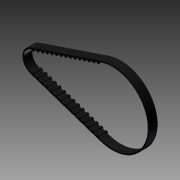
# Autodesk Inventor part: short turn belt
Saved by Autodesk Inventor 2012 (Build 160160000, 160)
## iProperties
Created: 2013-11-05
Part Number: short turn belt
Material: Default
Document SubType Name: Modeling
Designer: Bryce
Density: 1 g/cm^3
Author: Bryce
Autodesk Inventor part; units mm, degrees
ref_plane "YZ Plane" through (0, 0, 0) normal (1, 0, 0) x (0, 1, 0)
ref_plane "XZ Plane" through (0, 0, 0) normal (0, 1, 0) x (-1, 0, 0)
ref_plane "XY Plane" through (0, 0, 0) normal (0, 0, 1) x (1, 0, 0)
sketch "Sketch1" plane through (0, 0, 0) normal (0, 0, 1) x (1, 0, 0)
  arc A0 (-3.6157, 10.7627) -> (-3.6157, -10.7627) centre (0, 0) ccw
  arc A1 (70.5622, -35.683) -> (70.5622, 35.683) centre (82.55, 0) ccw
  line L0 (-3.6157, 10.7627) -> (70.5622, 35.683)
  line L1 (-3.6157, -10.7627) -> (0.5217, -12.1527)
  arc A2 (70.1335, -36.9591) -> (70.1335, 36.9591) centre (82.55, 0) ccw
  line L2 (70.1335, -36.9591) -> (-4.0445, -12.0388)
  arc A3 (-4.0445, 12.0388) -> (-4.0445, -12.0388) centre (0, 0) ccw
  line L3 (-4.0445, 12.0388) -> (70.1335, 36.9591)
  arc A4 (0.1194, -11.4488) -> (-2.8701, -10.4444) centre (-1.4338, -11.1206) ccw
  arc A5 (-3.6157, -10.7627) -> (-2.8701, -10.4444) centre (-3.4216, -10.1848) ccw
  arc A6 (0.1194, -11.4488) -> (0.5217, -12.1527) centre (0.7159, -11.5748) ccw
  line L4 (0.5217, -12.1527) -> (70.5622, -35.683)
  line L5 (1.2961, -12.4128) -> (5.4336, -13.8028)
  arc A7 (5.0313, -13.0989) -> (2.0418, -12.0946) centre (3.4781, -12.7707) ccw
  arc A8 (1.2961, -12.4128) -> (2.0418, -12.0946) centre (1.4902, -11.835) ccw
  arc A9 (5.0313, -13.0989) -> (5.4336, -13.8028) centre (5.6277, -13.225) ccw
  line L6 (6.2079, -14.063) -> (10.3454, -15.453)
  arc A10 (9.9431, -14.7491) -> (6.9536, -13.7447) centre (8.3899, -14.4209) ccw
  arc A11 (6.2079, -14.063) -> (6.9536, -13.7447) centre (6.402, -13.4851) ccw
  arc A12 (9.9431, -14.7491) -> (10.3454, -15.453) centre (10.5395, -14.8751) ccw
  line L7 (11.1197, -15.7131) -> (15.2572, -17.1031)
  arc A13 (14.8549, -16.3992) -> (11.8654, -15.3949) centre (13.3017, -16.071) ccw
  arc A14 (11.1197, -15.7131) -> (11.8654, -15.3949) centre (11.3139, -15.1352) ccw
  arc A15 (14.8549, -16.3992) -> (15.2572, -17.1031) centre (15.4513, -16.5252) ccw
  line L8 (16.0315, -17.3632) -> (20.169, -18.7532)
  arc A16 (19.7667, -18.0493) -> (16.7772, -17.045) centre (18.2135, -17.7211) ccw
  arc A17 (16.0315, -17.3632) -> (16.7772, -17.045) centre (16.2257, -16.7854) ccw
  arc A18 (19.7667, -18.0493) -> (20.169, -18.7532) centre (20.3632, -18.1754) ccw
  line L9 (20.9434, -19.0134) -> (25.0809, -20.4034)
  arc A19 (24.6786, -19.6995) -> (21.689, -18.6952) centre (23.1254, -19.3713) ccw
  arc A20 (20.9434, -19.0134) -> (21.689, -18.6952) centre (21.1375, -18.4355) ccw
  arc A21 (24.6786, -19.6995) -> (25.0809, -20.4034) centre (25.275, -19.8255) ccw
  line L10 (25.8552, -20.6635) -> (29.9927, -22.0535)
  arc A22 (29.5904, -21.3496) -> (26.6009, -20.3453) centre (28.0372, -21.0214) ccw
  arc A23 (25.8552, -20.6635) -> (26.6009, -20.3453) centre (26.0493, -20.0857) ccw
  arc A24 (29.5904, -21.3496) -> (29.9927, -22.0535) centre (30.1868, -21.4757) ccw
  line L11 (30.767, -22.3137) -> (34.9045, -23.7037)
  arc A25 (34.5022, -22.9998) -> (31.5127, -21.9954) centre (32.949, -22.6716) ccw
  arc A26 (30.767, -22.3137) -> (31.5127, -21.9954) centre (30.9612, -21.7358) ccw
  arc A27 (34.5022, -22.9998) -> (34.9045, -23.7037) centre (35.0986, -23.1258) ccw
  line L12 (35.6788, -23.9638) -> (39.8163, -25.3538)
  arc A28 (39.414, -24.6499) -> (36.4245, -23.6456) centre (37.8608, -24.3217) ccw
  arc A29 (35.6788, -23.9638) -> (36.4245, -23.6456) centre (35.873, -23.3859) ccw
  arc A30 (39.414, -24.6499) -> (39.8163, -25.3538) centre (40.0105, -24.7759) ccw
  line L13 (40.5907, -25.6139) -> (44.7282, -27.0039)
  arc A31 (44.3259, -26.3) -> (41.3363, -25.2957) centre (42.7727, -25.9719) ccw
  arc A32 (40.5907, -25.6139) -> (41.3363, -25.2957) centre (40.7848, -25.0361) ccw
  arc A33 (44.3259, -26.3) -> (44.7282, -27.0039) centre (44.9223, -26.4261) ccw
  line L14 (45.5025, -27.2641) -> (49.64, -28.6541)
  arc A34 (49.2377, -27.9502) -> (46.2482, -26.9459) centre (47.6845, -27.622) ccw
  arc A35 (45.5025, -27.2641) -> (46.2482, -26.9459) centre (45.6966, -26.6862) ccw
  arc A36 (49.2377, -27.9502) -> (49.64, -28.6541) centre (49.8341, -28.0762) ccw
  line L15 (50.4143, -28.9142) -> (54.5518, -30.3042)
  arc A37 (54.1495, -29.6003) -> (51.16, -28.596) centre (52.5963, -29.2721) ccw
  arc A38 (50.4143, -28.9142) -> (51.16, -28.596) centre (50.6085, -28.3364) ccw
  arc A39 (54.1495, -29.6003) -> (54.5518, -30.3042) centre (54.7459, -29.7264) ccw
  line L16 (55.3261, -30.5644) -> (59.4636, -31.9544)
  arc A40 (59.0613, -31.2505) -> (56.0718, -30.2461) centre (57.5081, -30.9223) ccw
  arc A41 (55.3261, -30.5644) -> (56.0718, -30.2461) centre (55.5203, -29.9865) ccw
  arc A42 (59.0613, -31.2505) -> (59.4636, -31.9544) centre (59.6578, -31.3765) ccw
  line L17 (60.238, -32.2145) -> (64.3755, -33.6045)
  arc A43 (63.9732, -32.9006) -> (60.9836, -31.8963) centre (62.42, -32.5724) ccw
  arc A44 (60.238, -32.2145) -> (60.9836, -31.8963) centre (60.4321, -31.6366) ccw
  arc A45 (63.9732, -32.9006) -> (64.3755, -33.6045) centre (64.5696, -33.0266) ccw
  line L18 (65.1498, -33.8646) -> (69.2873, -35.2546)
  arc A46 (68.885, -34.5507) -> (65.8955, -33.5464) centre (67.3318, -34.2226) ccw
  arc A47 (65.1498, -33.8646) -> (65.8955, -33.5464) centre (65.3439, -33.2868) ccw
  arc A48 (68.885, -34.5507) -> (69.2873, -35.2546) centre (69.4814, -34.6768) ccw
  line L19 (0, 0) -> (82.55, 0) construction
  line L20 (-3.6157, 10.7627) -> (0.5217, 12.1527)
  arc A49 (-2.8701, 10.4444) -> (0.1194, 11.4488) centre (-1.4338, 11.1206) ccw
  arc A50 (-2.8701, 10.4444) -> (-3.6157, 10.7627) centre (-3.4216, 10.1848) ccw
  arc A51 (0.5217, 12.1527) -> (0.1194, 11.4488) centre (0.7159, 11.5748) ccw
  line L21 (1.2961, 12.4128) -> (5.4336, 13.8028)
  arc A52 (2.0418, 12.0946) -> (5.0313, 13.0989) centre (3.4781, 12.7707) ccw
  arc A53 (2.0418, 12.0946) -> (1.2961, 12.4128) centre (1.4902, 11.835) ccw
  arc A54 (5.4336, 13.8028) -> (5.0313, 13.0989) centre (5.6277, 13.225) ccw
  line L22 (6.2079, 14.063) -> (10.3454, 15.453)
  arc A55 (6.9536, 13.7447) -> (9.9431, 14.7491) centre (8.3899, 14.4209) ccw
  arc A56 (6.9536, 13.7447) -> (6.2079, 14.063) centre (6.402, 13.4851) ccw
  arc A57 (10.3454, 15.453) -> (9.9431, 14.7491) centre (10.5395, 14.8751) ccw
  line L23 (11.1197, 15.7131) -> (15.2572, 17.1031)
  arc A58 (11.8654, 15.3949) -> (14.8549, 16.3992) centre (13.3017, 16.071) ccw
  arc A59 (11.8654, 15.3949) -> (11.1197, 15.7131) centre (11.3139, 15.1352) ccw
  arc A60 (15.2572, 17.1031) -> (14.8549, 16.3992) centre (15.4513, 16.5252) ccw
  line L24 (16.0315, 17.3632) -> (20.169, 18.7532)
  arc A61 (16.7772, 17.045) -> (19.7667, 18.0493) centre (18.2135, 17.7211) ccw
  arc A62 (16.7772, 17.045) -> (16.0315, 17.3632) centre (16.2257, 16.7854) ccw
  arc A63 (20.169, 18.7532) -> (19.7667, 18.0493) centre (20.3632, 18.1754) ccw
  line L25 (20.9434, 19.0134) -> (25.0809, 20.4034)
  arc A64 (21.689, 18.6952) -> (24.6786, 19.6995) centre (23.1254, 19.3713) ccw
  arc A65 (21.689, 18.6952) -> (20.9434, 19.0134) centre (21.1375, 18.4355) ccw
  arc A66 (25.0809, 20.4034) -> (24.6786, 19.6995) centre (25.275, 19.8255) ccw
  line L26 (25.8552, 20.6635) -> (29.9927, 22.0535)
  arc A67 (26.6009, 20.3453) -> (29.5904, 21.3496) centre (28.0372, 21.0214) ccw
  arc A68 (26.6009, 20.3453) -> (25.8552, 20.6635) centre (26.0493, 20.0857) ccw
  arc A69 (29.9927, 22.0535) -> (29.5904, 21.3496) centre (30.1868, 21.4757) ccw
  line L27 (30.767, 22.3137) -> (34.9045, 23.7037)
  arc A70 (31.5127, 21.9954) -> (34.5022, 22.9998) centre (32.949, 22.6716) ccw
  arc A71 (31.5127, 21.9954) -> (30.767, 22.3137) centre (30.9612, 21.7358) ccw
  arc A72 (34.9045, 23.7037) -> (34.5022, 22.9998) centre (35.0986, 23.1258) ccw
  line L28 (35.6788, 23.9638) -> (39.8163, 25.3538)
  arc A73 (36.4245, 23.6456) -> (39.414, 24.6499) centre (37.8608, 24.3217) ccw
  arc A74 (36.4245, 23.6456) -> (35.6788, 23.9638) centre (35.873, 23.3859) ccw
  arc A75 (39.8163, 25.3538) -> (39.414, 24.6499) centre (40.0105, 24.7759) ccw
  line L29 (40.5907, 25.6139) -> (44.7282, 27.0039)
  arc A76 (41.3363, 25.2957) -> (44.3259, 26.3) centre (42.7727, 25.9719) ccw
  arc A77 (41.3363, 25.2957) -> (40.5907, 25.6139) centre (40.7848, 25.0361) ccw
  arc A78 (44.7282, 27.0039) -> (44.3259, 26.3) centre (44.9223, 26.4261) ccw
  line L30 (45.5025, 27.2641) -> (49.64, 28.6541)
  arc A79 (46.2482, 26.9459) -> (49.2377, 27.9502) centre (47.6845, 27.622) ccw
  arc A80 (46.2482, 26.9459) -> (45.5025, 27.2641) centre (45.6966, 26.6862) ccw
  arc A81 (49.64, 28.6541) -> (49.2377, 27.9502) centre (49.8341, 28.0762) ccw
  line L31 (50.4143, 28.9142) -> (54.5518, 30.3042)
  arc A82 (51.16, 28.596) -> (54.1495, 29.6003) centre (52.5963, 29.2721) ccw
  arc A83 (51.16, 28.596) -> (50.4143, 28.9142) centre (50.6085, 28.3364) ccw
  arc A84 (54.5518, 30.3042) -> (54.1495, 29.6003) centre (54.7459, 29.7264) ccw
  line L32 (55.3261, 30.5644) -> (59.4636, 31.9544)
  arc A85 (56.0718, 30.2461) -> (59.0613, 31.2505) centre (57.5081, 30.9223) ccw
  arc A86 (56.0718, 30.2461) -> (55.3261, 30.5644) centre (55.5203, 29.9865) ccw
  arc A87 (59.4636, 31.9544) -> (59.0613, 31.2505) centre (59.6578, 31.3765) ccw
  line L33 (60.238, 32.2145) -> (64.3755, 33.6045)
  arc A88 (60.9836, 31.8963) -> (63.9732, 32.9006) centre (62.42, 32.5724) ccw
  arc A89 (60.9836, 31.8963) -> (60.238, 32.2145) centre (60.4321, 31.6366) ccw
  arc A90 (64.3755, 33.6045) -> (63.9732, 32.9006) centre (64.5696, 33.0266) ccw
  line L34 (65.1498, 33.8646) -> (69.2873, 35.2546)
  arc A91 (65.8955, 33.5464) -> (68.885, 34.5507) centre (67.3318, 34.2226) ccw
  arc A92 (65.8955, 33.5464) -> (65.1498, 33.8646) centre (65.3439, 33.2868) ccw
  arc A93 (69.2873, 35.2546) -> (68.885, 34.5507) centre (69.4814, 34.6768) ccw
  line L35 (-3.4216, -10.1848) -> (0.7159, -11.5748) construction
  dimension "d0" = 82.55
  dimension "d1" = 11.3538
  dimension "d2" = 12.7
  dimension "d4" = 1.5875
  dimension "d5" = 0.6096
  dimension "d9" = 5.1816
  dimension "d16" = 37.6428
  dimension "d17" = 0.254
  constraints: 188 point on circle, 104 symmetric about line, 94 centre point, 72 end point, 15 tangent, 1 coincident, 1 equal radius, 1 horizontal alignment, 201 other
  measures "d0" distance of L19.end point (0, 0)
  measures "d1" radius of A0
  measures "d2" radius of A3
  measures "d4" radius of A4
  measures "d5" radius of A5
  measures "d9" distance of L1.start L5.start
  measures "d16" radius of A1
  measures "d17" distance from line of A4.centre L35
extrude "Extrusion1" add sketch "Sketch1" along normal blind 9 contours L0 A51 A49 A50 | A5 A4 A6 L1 | L0 A54 A52 A53 | A8 A7 A9 L4 | L0 A57 A55 A56 | A11 A10 A12 L4 | L0 A60 A58 A59 | A14 A13 A15 L4 | L0 A63 A61 A62 | A17 A16 A18 L4 | L0 A66 A64 A65 | A20 A19 A21 L4 | L0 A69 A67 A68 | A23 A22 A24 L4 | L0 A72 A70 A71 | A26 A25 A27 L4 | L0 A75 A73 A74 | A29 A28 A30 L4 | L0 A78 A76 A77 | A32 A31 A33 L4 | L0 A81 A79 A80 | A35 A34 A36 L4 | L0 A84 A82 A83 | A38 A37 A39 L4 | L0 A87 A85 A86 | A41 A40 A42 L4 | L0 A90 A88 A89 | A44 A43 A45 L4 | L0 A93 A91 A92 | A47 A46 A48 L4 | L2 A3 L3 A2
body "Solid1"
